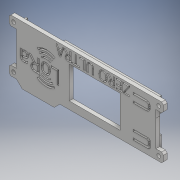
# Autodesk Inventor part: ttgo_lora_oled_case_lid
Saved by Autodesk Inventor 2017 (Build 210142000, 142)
## iProperties
Created: 2021-11-16
Part Number: ttgo_lora_oled_case_lid
Material: Generic
Document SubType Name: Modeling
Designer: simulator
Density: 1 g/cm^3
Appearance: Default
Author: simulator
Autodesk Inventor part; units mm, degrees
ref_plane "YZ Plane" through (0, 0, 0) normal (1, 0, 0) x (0, 1, 0)
ref_plane "XZ Plane" through (0, 0, 0) normal (0, 1, 0) x (-1, 0, 0)
ref_plane "XY Plane" through (0, 0, 0) normal (0, 0, 1) x (1, 0, 0)
sketch "Sketch1" plane through (0, 0, 0) normal (0, 1, 0) x (-1, 0, 0)
  circle A0 centre (-53.5, -14.5) radius 1
  circle A1 centre (23.5, -14.5) radius 1
  circle A2 centre (23.5, 8.5) radius 1
  circle A3 centre (-53.5, 8.5) radius 1
  line L0 (-51, -16) -> (-51, -8)
  line L1 (-51, -8) -> (-52, -8)
  line L2 (-52, -8) -> (-52, -12)
  line L3 (-55, -12) -> (-52, -12)
  line L4 (-56, -13) -> (-55, -12)
  line L5 (-56, -16) -> (-56, -13)
  line L6 (-55, -17) -> (-56, -16)
  line L7 (-1, -17) -> (-55, -17)
  line L8 (-1, -17) -> (2, -20)
  line L9 (2, -20) -> (19, -20)
  line L10 (19, -20) -> (22, -17)
  line L11 (22, -17) -> (25, -17)
  line L12 (25, -17) -> (26, -16)
  line L13 (26, -16) -> (26, -13)
  line L14 (26, -13) -> (25, -12)
  line L15 (25, -12) -> (22, -12)
  line L16 (22, -12) -> (22, 6)
  line L17 (25, 6) -> (22, 6)
  line L18 (26, 7) -> (25, 6)
  line L19 (26, 10) -> (26, 7)
  line L20 (25, 11) -> (26, 10)
  line L21 (-55, 11) -> (25, 11)
  line L22 (-55, 11) -> (-56, 10)
  line L23 (-56, 10) -> (-56, 7)
  line L24 (-56, 7) -> (-55, 6)
  line L25 (-55, 6) -> (-52, 6)
  line L26 (-52, 6) -> (-52, 2)
  line L27 (-52, 2) -> (-51, 2)
  line L28 (-51, 2) -> (-51, 10)
  line L29 (-51, 10) -> (0, 10)
  line L30 (0, 10) -> (0, 2)
  line L31 (0, 2) -> (2.5, 2)
  line L32 (2.5, 2) -> (2.5, 10)
  line L33 (2.5, 10) -> (21, 10)
  line L34 (21, 10) -> (21, -16)
  line L35 (21, -16) -> (2.5, -16)
  line L36 (2.5, -16) -> (2.5, -8)
  line L37 (2.5, -8) -> (0, -8)
  line L38 (0, -8) -> (0, -16)
  line L39 (0, -16) -> (-51, -16)
  point P0 (0, 0)
  point P1 (0, 0)
  constraints: 80 end point, 4 centre point
sketch "Sketch2" plane through (0, 0, 0) normal (0, 1, 0) x (-1, 0, 0)
  line L0 (-33, 2) -> (-33, -13)
  line L1 (-33, -13) -> (-8, -13)
  line L2 (-40, -14) -> (-49, -14)
  line L3 (-49, -9) -> (-40, -9)
  line L4 (-49, -14) -> (-49, -9)
  line L5 (19, -20) -> (2, -20)
  line L6 (-8, -13) -> (-8, 2)
  line L7 (22, -12) -> (22, 6) projected
  line L8 (22, -17) -> (25, -17) projected
  line L9 (25, -17) -> (26, -16) projected
  line L10 (26, -16) -> (26, -13) projected
  line L11 (25, -12) -> (22, -12) projected
  line L12 (-55, -12) -> (-52, -12)
  circle A0 centre (-53.5, -14.5) radius 1
  line L13 (-52, 2) -> (-52, -12)
  line L14 (-52, 6) -> (-52, 2)
  line L15 (-55, 6) -> (-52, 6)
  circle A1 centre (-53.5, 8.5) radius 1
  line L16 (-1, -17) -> (-55, -17)
  line L17 (-55, 11) -> (25, 11)
  circle A2 centre (23.5, 8.5) radius 1
  circle A3 centre (23.5, -14.5) radius 1
  line L18 (-55, -17) -> (-56, -16)
  line L19 (-56, -16) -> (-56, -13)
  line L20 (-56, -13) -> (-55, -12)
  line L21 (-1, -17) -> (2, -20)
  line L22 (2, -20) -> (19, -20)
  line L23 (22, -12) -> (22, 6)
  line L24 (25, 11) -> (26, 10)
  line L25 (26, 10) -> (26, 7)
  line L26 (25, 6) -> (22, 6)
  line L27 (26, 7) -> (25, 6)
  line L28 (19, -20) -> (22, -17)
  line L29 (25, -12) -> (22, -12)
  line L30 (26, -13) -> (25, -12)
  line L31 (22, -17) -> (25, -17)
  line L32 (26, -16) -> (26, -13)
  line L33 (25, -17) -> (26, -16)
  line L34 (-55, 11) -> (-56, 10)
  line L35 (-56, 7) -> (-55, 6)
  line L36 (-56, 10) -> (-56, 7)
  line L37 (-8, 2) -> (-33, 2)
  arc A4 (-52, 1) -> (-52, 2) centre (-420844.4746, 2.0039) ccw
  line L38 (-40, -8) -> (-40, -15)
  line L39 (-38, -13) -> (-48, -13)
  line L40 (-48, -13) -> (-48, -10)
  line L41 (-48, -10) -> (-38, -10)
  line L42 (-38, -10) -> (-38, -13)
  line L43 (22, -3) -> (-52, -3)
  line L44 (-40, -14) -> (-49, -14)
  line L45 (-49, -14) -> (-49, -13)
  line L46 (-49, -13) -> (-40, -13)
  line L47 (-40, -13) -> (-40, -14)
  line L48 (-49, -9) -> (-48, -9)
  line L49 (-48, -9) -> (-48, -14)
  line L50 (-48, -14) -> (-49, -14)
  line L51 (-49, -14) -> (-49, -9)
  line L52 (-49, -9) -> (-40, -9)
  line L53 (-40, -9) -> (-40, -10)
  line L54 (-40, -10) -> (-49, -10)
  line L55 (-49, -10) -> (-49, -9)
  line L56 (-40, -9) -> (-39, -9)
  line L57 (-39, -9) -> (-39, -10)
  line L58 (-39, -10) -> (-40, -10)
  line L59 (-40, -10) -> (-40, -9)
  line L60 (-40, -14) -> (-39, -14)
  line L61 (-39, -14) -> (-39, -13)
  line L62 (-39, -13) -> (-40, -13)
  line L63 (-40, -13) -> (-40, -14)
  line L64 (-49, 3) -> (-40, 3)
  line L65 (-49, 8) -> (-49, 3)
  line L66 (-40, 8) -> (-49, 8)
  line L67 (-40, 2) -> (-40, 9)
  line L68 (-38, 7) -> (-48, 7)
  line L69 (-48, 7) -> (-48, 4)
  line L70 (-48, 4) -> (-38, 4)
  line L71 (-38, 4) -> (-38, 7)
  line L72 (-40, 8) -> (-49, 8)
  line L73 (-49, 8) -> (-49, 7)
  line L74 (-49, 7) -> (-40, 7)
  line L75 (-40, 7) -> (-40, 8)
  line L76 (-49, 3) -> (-48, 3)
  line L77 (-48, 3) -> (-48, 8)
  line L78 (-48, 8) -> (-49, 8)
  line L79 (-49, 8) -> (-49, 3)
  line L80 (-49, 3) -> (-40, 3)
  line L81 (-40, 3) -> (-40, 4)
  line L82 (-40, 4) -> (-49, 4)
  line L83 (-49, 4) -> (-49, 3)
  line L84 (-40, 3) -> (-39, 3)
  line L85 (-39, 3) -> (-39, 4)
  line L86 (-39, 4) -> (-40, 4)
  line L87 (-40, 4) -> (-40, 3)
  line L88 (-40, 8) -> (-39, 8)
  line L89 (-39, 8) -> (-39, 7)
  line L90 (-39, 7) -> (-40, 7)
  line L91 (-40, 7) -> (-40, 8)
  point P0 (-56, 8.5)
  point P1 (-56, -14.5)
  point P2 (-48, -11.5)
  point P3 (-48, -11.5)
  point P4 (-48, 5.5)
  point P5 (-48, 5.5)
  dimension "d1" = 5
  dimension "d2" = 10
  dimension "d3" = 3
  dimension "d4" = 1
  constraints: 174 end point, 27 symmetric about line, 17 point on line, 12 parallel, 11 horizontal, 7 perpendicular, 5 centre point, 3 midpoint, 3 vertical, 2 point on circle, 1 tangent, 7 other
  measures "d1" distance of L4.start L3.start
  measures "d2" distance of L40.end L41.end
  measures "d3" distance of L39.end L40.end
  measures "d4" distance from line of point (-48, -11.5) L4
extrude "Extrusion1" add sketch "Sketch2" along normal blind 2 contours L0 L43 L13 L14 L15 L35 L36 L34 L17 L24 L25 L27 L26 L7 L6 L37 | L0 L1 L6 L43 L7 L11 L30 L10 L9 L8 L28 L5 L21 L16 L18 L19 L20 L12 L13 | L38 L39 L61 L60 | L39 L40 L41 L38 | L38 L41 L42 L39 | L38 L56 L57 L41 | L67 L70 L85 L84 | L69 L68 L67 L70 | L67 L68 L71 L70 | L67 L88 L89 L68
sketch "Sketch3" plane through (0, 2, 0) normal (0, 1, 0) x (1, 0, 0)
  circle A0 centre (53.5, 14.5) radius 1
  circle A1 centre (-23.5, 14.5) radius 1
  circle A2 centre (-23.5, -8.5) radius 1
  circle A3 centre (53.5, -8.5) radius 1
  line L0 (51, 16) -> (51, 8)
  line L1 (51, 8) -> (52, 8)
  line L2 (52, 8) -> (52, 12)
  line L3 (55, 12) -> (52, 12)
  line L4 (56, 13) -> (55, 12)
  line L5 (56, 16) -> (56, 13)
  line L6 (55, 17) -> (56, 16)
  line L7 (1, 17) -> (55, 17)
  line L8 (1, 17) -> (-2, 20)
  line L9 (-2, 20) -> (-19, 20)
  line L10 (-19, 20) -> (-22, 17)
  line L11 (-22, 17) -> (-25, 17)
  line L12 (-25, 17) -> (-26, 16)
  line L13 (-26, 16) -> (-26, 13)
  line L14 (-26, 13) -> (-25, 12)
  line L15 (-25, 12) -> (-22, 12)
  line L16 (-22, 12) -> (-22, -6)
  line L17 (-25, -6) -> (-22, -6)
  line L18 (-26, -7) -> (-25, -6)
  line L19 (-26, -10) -> (-26, -7)
  line L20 (-25, -11) -> (-26, -10)
  line L21 (55, -11) -> (-25, -11)
  line L22 (55, -11) -> (56, -10)
  line L23 (56, -10) -> (56, -7)
  line L24 (56, -7) -> (55, -6)
  line L25 (55, -6) -> (52, -6)
  line L26 (52, -6) -> (52, -2)
  line L27 (52, -2) -> (51, -2)
  line L28 (51, -2) -> (51, -10)
  line L29 (51, -10) -> (0, -10)
  line L30 (0, -10) -> (0, -2)
  line L31 (0, -2) -> (-2.5, -2)
  line L32 (-2.5, -2) -> (-2.5, -10)
  line L33 (-2.5, -10) -> (-21, -10)
  line L34 (-21, -10) -> (-21, 16)
  line L35 (-21, 16) -> (-2.5, 16)
  line L36 (-2.5, 16) -> (-2.5, 8)
  line L37 (-2.5, 8) -> (0, 8)
  line L38 (0, 8) -> (0, 16)
  line L39 (0, 16) -> (51, 16)
  circle A4 centre (-23.5, 14.5) radius 1 projected
  line L40 (0, 16) -> (51, 16)
  line L41 (51, 16) -> (51, 15)
  line L42 (51, 15) -> (0, 15)
  line L43 (0, 15) -> (0, 16)
  line L44 (0, -10) -> (51, -10)
  line L45 (51, -10) -> (51, -9)
  line L46 (51, -9) -> (0, -9)
  line L47 (0, -9) -> (0, -10)
  line L48 (-21, 16) -> (-20, 16)
  line L49 (-20, 16) -> (-20, -10)
  line L50 (-20, -10) -> (-21, -10)
  line L51 (-21, -10) -> (-21, 16)
  line L52 (51, -2) -> (50, -2)
  line L53 (50, -2) -> (50, -10)
  line L54 (50, -10) -> (51, -10)
  line L55 (51, -10) -> (51, -2)
  line L56 (51, 8) -> (50, 8)
  line L57 (50, 8) -> (50, 16)
  line L58 (50, 16) -> (51, 16)
  line L59 (51, 16) -> (51, 8)
  point P0 (0, 0)
  point P1 (0, 0)
  dimension "d8" = 1
  dimension "d9" = 1
  dimension "d10" = 1
  dimension "d11" = 1
  constraints: 120 end point, 10 parallel, 6 point on line, 5 horizontal, 5 perpendicular, 4 centre point
  measures "d8" distance of L40.end L41.end
  measures "d9" distance of L45.end L44.end
  measures "d10" distance of L49.end L50.end
  measures "d11" distance of L54.end L53.end
extrude "Extrusion2" add sketch "Sketch3" along normal blind 2 contours L0 L42 L57 L39 | L0 L56 L57 L42 | L57 L42 L38 L39 | L49 L33 L34 L35 | L46 L53 L29 L30 | L53 L52 L28 L46 | L46 L28 L29 L53
chamfer "Chamfer1" distance 1 angle 45 3 edges at (-20, 2, -3) (25, 2, -15) (25, 2, 9)
fillet "Fillet1" radius 1 3 edges at (48, 1, -13) (48, 1, 4) (48, 1, 7)
fillet "Fillet2" radius 1 3 edges at (49, 1, -14) (49, 1, -9) (48, 1, -10)
sketch "Sketch4" plane through (0, 0, 0) normal (0, -1, 0) x (1, 0, 0)
  line L0 (48, -14) -> (40, -14) projected
  line L1 (40, -13) -> (40, -14) projected
  line L2 (47, -13) -> (40, -13) projected
  arc A0 (47, -13) -> (48, -12) centre (47, -12) ccw projected
  line L3 (48, -12) -> (48, -11) projected
  line L4 (47, -10) -> (40, -10) projected
  line L5 (40, -10) -> (40, -9) projected
  line L6 (40, -9) -> (48, -9) projected
  arc A1 (48, 6) -> (47, 7) centre (47, 6) ccw projected
  line L7 (47, 7) -> (40, 7) projected
  line L8 (40, 7) -> (40, 8) projected
  line L9 (40, 8) -> (49, 8) projected
  line L10 (49, 8) -> (49, 3) projected
  line L11 (49, 3) -> (40, 3) projected
  line L12 (40, 3) -> (40, 4) projected
  line L13 (40, 4) -> (47, 4) projected
  arc A2 (47, 4) -> (48, 5) centre (47, 5) ccw projected
  line L14 (48, 5) -> (48, 6) projected
  line L15 (-22, -17) -> (-19, -20) projected
  line L16 (-19, -20) -> (-2, -20) projected
  line L17 (-2, -20) -> (1, -17) projected
  line L18 (1, -17) -> (55, -17) projected
  line L19 (55, -17) -> (56, -16) projected
  line L20 (56, -16) -> (56, -13) projected
  line L21 (56, -13) -> (55, -12) projected
  line L22 (55, -12) -> (52, -12) projected
  line L23 (52, -12) -> (52, 2) projected
  line L24 (52, 2) -> (52, 6) projected
  line L25 (52, 6) -> (55, 6) projected
  line L26 (55, 6) -> (56, 7) projected
  line L27 (56, 7) -> (56, 10) projected
  line L28 (56, 10) -> (55, 11) projected
  line L29 (55, 11) -> (-25, 11) projected
  line L30 (-25, 11) -> (-26, 10) projected
  line L31 (-26, 10) -> (-26, 7) projected
  line L32 (-26, 7) -> (-25, 6) projected
  line L33 (-25, 6) -> (-22, 6) projected
  line L34 (-22, 6) -> (-22, -12) projected
  line L35 (-22, -12) -> (-25, -12) projected
  line L36 (-25, -12) -> (-26, -13) projected
  line L37 (-26, -13) -> (-26, -16) projected
  line L38 (-26, -16) -> (-25, -17) projected
  line L39 (-25, -17) -> (-22, -17) projected
  circle A3 centre (53.5, -14.5) radius 1 projected
  circle A4 centre (53.5, 8.5) radius 1 projected
  circle A5 centre (-23.5, 8.5) radius 1 projected
  circle A6 centre (-23.5, -14.5) radius 1 projected
  line L40 (33, 2) -> (33, -13) projected
  line L41 (33, -13) -> (8, -13) projected
  line L42 (8, -13) -> (8, 2) projected
  line L43 (8, 2) -> (33, 2) projected
  line L44 (33, 2) -> (8, 2)
  line L45 (8, 2) -> (8, 4)
  line L46 (8, 4) -> (33, 4)
  line L47 (33, 4) -> (33, 2)
  line L48 (8, -13) -> (6, -13)
  line L49 (6, -13) -> (6, 4)
  line L50 (6, 4) -> (8, 4)
  line L51 (8, 4) -> (8, -13)
  arc A7 (48, -11) -> (47, -10) centre (47, -11) ccw projected
  arc A8 (49, -10) -> (48, -9) centre (48, -10) ccw projected
  line L52 (49, -10) -> (49, -13) projected
  arc A9 (48, -14) -> (49, -13) centre (48, -13) ccw projected
  point P0 (0, 0)
  dimension "d19" = 2
  dimension "d20" = 2
  constraints: 16 end point, 4 parallel, 2 horizontal, 2 perpendicular, 1 point on line
  measures "d19" distance of L44.end L45.end
  measures "d20" distance of L49.end L50.end
extrude "Extrusion3" cut sketch "Sketch4" against normal blind 10 contours L43 L45 L46 L47 | L42 L48 L49 L50 L45
fillet "Fillet3" radius 2 2 edges at (49, 1, 8) (49, 1, 3)
sketch "Sketch5" plane through (0, 0, 0) normal (0, -1, 0) x (1, 0, 0)
  line L0 (1.2295, -8.816) -> (-31.2797, -8.816) construction
  line L1 (-31.2797, -8.816) -> (-31.2797, 0.8087) construction
  line L2 (-31.2797, 0.8087) -> (1.2295, 0.8087) construction
  line L3 (1.2295, 0.8087) -> (1.2295, -8.816) construction
  line L4 (-3.9903, -0.4302) -> (-3.6005, 0.1309)
  line L5 (-3.0082, 0.9561) -> (-2.5783, 1.563)
  line L6 (-2.0871, 2.2564) -> (-1.495, 3.0924)
  arc A0 (-3.9903, -0.4302) -> (-8.565, -0.5063) centre (-6.2185, -4.0213) ccw
  arc A1 (-8.6056, -7.5089) -> (-4.0659, -7.6583) centre (-6.2185, -4.0213) ccw
  arc A2 (-3.6005, 0.1309) -> (-8.9501, 0.0571) centre (-6.2185, -4.0213) ccw
  arc A3 (-8.9329, -7.9708) -> (-3.7378, -8.1216) centre (-6.2185, -4.0213) ccw
  line L7 (-8.565, -0.5063) -> (-8.9501, 0.0571)
  arc A4 (-3.0082, 0.9561) -> (-9.5252, 0.8926) centre (-6.2185, -4.0213) ccw
  arc A5 (-9.5865, -8.8935) -> (-3.0831, -9.0463) centre (-6.2185, -4.0213) ccw
  arc A6 (-2.5783, 1.563) -> (-9.9458, 1.5053) centre (-6.2185, -4.0213) ccw
  arc A7 (-10.016, -9.4999) -> (-2.6531, -9.6537) centre (-6.2185, -4.0213) ccw
  arc A8 (-2.0871, 2.2564) -> (-10.4264, 2.2054) centre (-6.2185, -4.0213) ccw
  arc A9 (-1.495, 3.0924) -> (-11.0059, 3.0495) centre (-6.2185, -4.0213) ccw
  line L8 (-9.5252, 0.8926) -> (-9.9458, 1.5053)
  line L9 (-10.4264, 2.2054) -> (-11.0059, 3.0495)
  line L10 (-4.0659, -7.6583) -> (-3.7378, -8.1216)
  line L11 (-2.6531, -9.6537) -> (-3.0831, -9.0463)
  line L12 (-2.1618, -10.3476) -> (-1.5696, -11.184)
  arc A10 (-11.9743, 0.8087) -> (-12.0038, -8.816) centre (-6.2185, -4.0213) ccw
  line L13 (-10.5069, -10.1929) -> (-11.0988, -11.0284)
  arc A11 (-13.2592, 0.8087) -> (-13.2833, -8.816) centre (-6.2185, -4.0213) ccw
  line L14 (-8.6056, -7.5089) -> (-8.9329, -7.9708)
  line L15 (-9.5865, -8.8935) -> (-10.016, -9.4999)
  arc A12 (-10.5069, -10.1929) -> (-2.1618, -10.3476) centre (-6.2185, -4.0213) ccw
  arc A13 (-0.4333, -8.816) -> (-0.4627, 0.8087) centre (-6.2185, -4.0213) ccw
  arc A14 (-11.0988, -11.0284) -> (-1.5696, -11.184) centre (-6.2185, -4.0213) ccw
  arc A15 (0.8463, -8.816) -> (0.8222, 0.8087) centre (-6.2185, -4.0213) ccw
  line L16 (38.3682, 4.8239) -> (-10.0254, 4.8239) construction
  line L17 (-10.0254, 4.8239) -> (-10.0254, 15.0346) construction
  line L18 (-10.0254, 15.0346) -> (38.3682, 15.0346) construction
  line L19 (38.3682, 15.0346) -> (38.3682, 4.8239) construction
  line L20 (34.6729, 9.9292) -> (38.1656, 9.9292)
  line L21 (38.1656, 9.9292) -> (38.1656, 9.3093)
  line L22 (38.1656, 9.3093) -> (35.4914, 5.5208)
  line L23 (35.4914, 5.5208) -> (38.0441, 5.5208)
  line L24 (38.0441, 5.5208) -> (38.0441, 4.9292)
  line L25 (38.0441, 4.9292) -> (34.7418, 4.9292)
  line L26 (34.7418, 4.9292) -> (34.7418, 5.5289)
  line L27 (34.7418, 5.5289) -> (37.4444, 9.3377)
  line L28 (37.4444, 9.3377) -> (34.6729, 9.3377)
  line L29 (34.6729, 9.3377) -> (34.6729, 9.9292)
  line L30 (34.0165, 9.9292) -> (34.0165, 4.9292)
  line L31 (34.0165, 4.9292) -> (30.8885, 4.9292)
  line L32 (30.8885, 4.9292) -> (30.8885, 5.5208)
  line L33 (30.8885, 5.5208) -> (33.352, 5.5208)
  line L34 (33.352, 5.5208) -> (33.352, 6.8903)
  line L35 (33.352, 6.8903) -> (31.0546, 6.8903)
  line L36 (31.0546, 6.8903) -> (31.0546, 7.4819)
  line L37 (31.0546, 7.4819) -> (33.352, 7.4819)
  line L38 (33.352, 7.4819) -> (33.352, 9.3377)
  line L39 (33.352, 9.3377) -> (30.8885, 9.3377)
  line L40 (30.8885, 9.3377) -> (30.8885, 9.9292)
  line L41 (30.8885, 9.9292) -> (34.0165, 9.9292)
  line L42 (26.2896, 9.9292) -> (27.1527, 9.9292)
  line L43 (27.1527, 9.9292) -> (28.7329, 7.9398)
  line L44 (28.7329, 7.9398) -> (29.4946, 7.9398)
  line L45 (29.4946, 7.9398) -> (29.4946, 9.9292)
  line L46 (29.4946, 9.9292) -> (30.1591, 9.9292)
  line L47 (30.1591, 9.9292) -> (30.1591, 4.9292)
  line L48 (30.1591, 4.9292) -> (28.8707, 4.9292)
  spline S0 degree 2 poles (28.8707, 4.9292) (28.4412, 4.9292) (27.8617, 5.0224) (27.5984, 5.1926) knots 0 0 0 1 2 2 2
  spline S1 degree 2 poles (27.5984, 5.1926) (27.335, 5.3628) (27.0311, 5.8936) (27.0311, 6.2866) knots 0 0 0 1 2 2 2
  spline S2 degree 2 poles (27.0311, 6.2866) (27.0311, 6.8336) (27.5903, 7.5751) (28.0684, 7.7534) knots 0 0 0 1 2 2 2
  line L49 (28.0684, 7.7534) -> (26.2896, 9.9292)
  spline S3 degree 2 poles (27.724, 6.3393) (27.724, 6.1205) (27.8779, 5.7842) (28.04, 5.6748) knots 0 0 0 1 2 2 2
  spline S4 degree 2 poles (28.04, 5.6748) (28.1818, 5.5816) (28.5587, 5.5046) (28.8342, 5.5046) knots 0 0 0 1 2 2 2
  line L50 (28.8342, 5.5046) -> (29.4946, 5.5046)
  line L51 (29.4946, 5.5046) -> (29.4946, 7.3847)
  line L52 (29.4946, 7.3847) -> (28.9112, 7.3847)
  spline S5 degree 2 poles (28.9112, 7.3847) (28.6235, 7.3847) (28.1656, 7.2834) (28.0076, 7.1254) knots 0 0 0 1 2 2 2
  spline S6 degree 2 poles (28.0076, 7.1254) (27.8617, 6.9876) (27.724, 6.5986) (27.724, 6.3393) knots 0 0 0 1 2 2 2
  spline S7 degree 2 poles (22.3553, 5.5006) (22.0716, 5.8328) (21.7556, 6.8053) (21.7556, 7.4292) knots 0 0 0 1 2 2 2
  spline S8 degree 2 poles (21.7556, 7.4292) (21.7556, 8.037) (22.0635, 9.0216) (22.3553, 9.3539) knots 0 0 0 1 2 2 2
  spline S9 degree 2 poles (22.3553, 9.3539) (22.6632, 9.7023) (23.4776, 10.0346) (23.9679, 10.0346) knots 0 0 0 1 2 2 2
  spline S10 degree 2 poles (23.9679, 10.0346) (24.4744, 10.0346) (25.2848, 9.6902) (25.5805, 9.3539) knots 0 0 0 1 2 2 2
  spline S11 degree 2 poles (25.5805, 9.3539) (25.8682, 9.0216) (26.1762, 8.0451) (26.1762, 7.4292) knots 0 0 0 1 2 2 2
  spline S12 degree 2 poles (26.1762, 7.4292) (26.1762, 6.8012) (25.8642, 5.845) (25.5765, 5.5006) knots 0 0 0 1 2 2 2
  spline S13 degree 2 poles (25.5765, 5.5006) (25.2848, 5.1683) (24.4703, 4.8239) (23.9679, 4.8239) knots 0 0 0 1 2 2 2
  spline S14 degree 2 poles (23.9679, 4.8239) (23.4574, 4.8239) (22.6389, 5.1805) (22.3553, 5.5006) knots 0 0 0 1 2 2 2
  spline S15 degree 2 poles (22.4485, 7.4292) (22.4485, 6.9349) (22.6632, 6.1691) (22.8577, 5.9179) knots 0 0 0 1 2 2 2
  spline S16 degree 2 poles (22.8577, 5.9179) (23.0562, 5.6586) (23.6154, 5.3993) (23.9638, 5.3993) knots 0 0 0 1 2 2 2
  spline S17 degree 2 poles (23.9638, 5.3993) (24.3245, 5.3993) (24.8674, 5.6505) (25.0741, 5.9179) knots 0 0 0 1 2 2 2
  spline S18 degree 2 poles (25.0741, 5.9179) (25.2726, 6.1732) (25.4833, 6.943) (25.4833, 7.4292) knots 0 0 0 1 2 2 2
  spline S19 degree 2 poles (25.4833, 7.4292) (25.4833, 8.4139) (24.6567, 9.4592) (23.9638, 9.4592) knots 0 0 0 1 2 2 2
  spline S20 degree 2 poles (23.9638, 9.4592) (23.271, 9.4592) (22.4485, 8.4139) (22.4485, 7.4292) knots 0 0 0 1 2 2 2
  spline S21 degree 2 poles (17.1324, 10.0346) (17.5741, 10.0346) (18.2305, 9.8036) (18.4614, 9.5727) knots 0 0 0 1 2 2 2
  spline S22 degree 2 poles (18.4614, 9.5727) (18.7248, 9.3134) (18.9395, 8.584) (18.9395, 8.0492) knots 0 0 0 1 2 2 2
  line L53 (18.9395, 8.0492) -> (18.9395, 4.9292)
  line L54 (18.9395, 4.9292) -> (18.275, 4.9292)
  line L55 (18.275, 4.9292) -> (18.275, 8.0492)
  spline S23 degree 2 poles (18.275, 8.0492) (18.275, 8.3976) (18.1859, 8.8677) (18.0603, 9.0581) knots 0 0 0 1 2 2 2
  spline S24 degree 2 poles (18.0603, 9.0581) (17.9266, 9.2607) (17.4647, 9.4673) (17.1324, 9.4673) knots 0 0 0 1 2 2 2
  spline S25 degree 2 poles (17.1324, 9.4673) (16.8204, 9.4673) (16.3342, 9.2607) (16.2005, 9.0581) knots 0 0 0 1 2 2 2
  spline S26 degree 2 poles (16.2005, 9.0581) (16.0749, 8.8677) (15.9857, 8.4017) (15.9857, 8.0654) knots 0 0 0 1 2 2 2
  line L56 (15.9857, 8.0654) -> (15.9857, 4.9292)
  line L57 (15.9857, 4.9292) -> (15.3212, 4.9292)
  line L58 (15.3212, 4.9292) -> (15.3212, 8.0492)
  spline S27 degree 2 poles (15.3212, 8.0492) (15.3212, 8.5719) (15.5319, 9.3174) (15.7993, 9.5727) knots 0 0 0 1 2 2 2
  spline S28 degree 2 poles (15.7993, 9.5727) (16.0384, 9.8077) (16.6705, 10.0346) (17.1324, 10.0346) knots 0 0 0 1 2 2 2
  line L59 (11.472, 9.9292) -> (14.369, 9.9292)
  line L60 (14.369, 9.9292) -> (14.369, 4.9292)
  line L61 (14.369, 4.9292) -> (13.7045, 4.9292)
  line L62 (13.7045, 4.9292) -> (13.7045, 9.3377)
  line L63 (13.7045, 9.3377) -> (11.472, 9.3377)
  line L64 (11.472, 9.3377) -> (11.472, 9.9292)
  line L65 (9.7823, 9.9292) -> (9.7823, 5.5208)
  line L66 (9.7823, 5.5208) -> (11.4598, 5.5208)
  line L67 (11.4598, 5.5208) -> (11.4598, 4.9292)
  line L68 (11.4598, 4.9292) -> (7.4403, 4.9292)
  line L69 (7.4403, 4.9292) -> (7.4403, 5.5208)
  line L70 (7.4403, 5.5208) -> (9.1178, 5.5208)
  line L71 (9.1178, 5.5208) -> (9.1178, 9.9292)
  line L72 (9.1178, 9.9292) -> (9.7823, 9.9292)
  line L73 (3.0643, 9.9292) -> (3.9274, 9.9292)
  line L74 (3.9274, 9.9292) -> (5.5076, 7.9398)
  line L75 (5.5076, 7.9398) -> (6.2694, 7.9398)
  line L76 (6.2694, 7.9398) -> (6.2694, 9.9292)
  line L77 (6.2694, 9.9292) -> (6.9339, 9.9292)
  line L78 (6.9339, 9.9292) -> (6.9339, 4.9292)
  line L79 (6.9339, 4.9292) -> (5.6454, 4.9292)
  spline S29 degree 2 poles (5.6454, 4.9292) (5.2159, 4.9292) (4.6365, 5.0224) (4.3731, 5.1926) knots 0 0 0 1 2 2 2
  spline S30 degree 2 poles (4.3731, 5.1926) (4.1097, 5.3628) (3.8058, 5.8936) (3.8058, 6.2866) knots 0 0 0 1 2 2 2
  spline S31 degree 2 poles (3.8058, 6.2866) (3.8058, 6.8336) (4.365, 7.5751) (4.8431, 7.7534) knots 0 0 0 1 2 2 2
  line L80 (4.8431, 7.7534) -> (3.0643, 9.9292)
  spline S32 degree 2 poles (4.4987, 6.3393) (4.4987, 6.1205) (4.6527, 5.7842) (4.8147, 5.6748) knots 0 0 0 1 2 2 2
  spline S33 degree 2 poles (4.8147, 5.6748) (4.9566, 5.5816) (5.3334, 5.5046) (5.6089, 5.5046) knots 0 0 0 1 2 2 2
  line L81 (5.6089, 5.5046) -> (6.2694, 5.5046)
  line L82 (6.2694, 5.5046) -> (6.2694, 7.3847)
  line L83 (6.2694, 7.3847) -> (5.6859, 7.3847)
  spline S34 degree 2 poles (5.6859, 7.3847) (5.3982, 7.3847) (4.9403, 7.2834) (4.7823, 7.1254) knots 0 0 0 1 2 2 2
  spline S35 degree 2 poles (4.7823, 7.1254) (4.6365, 6.9876) (4.4987, 6.5986) (4.4987, 6.3393) knots 0 0 0 1 2 2 2
  line L84 (3.2062, 9.9292) -> (1.5206, 4.9292)
  line L85 (1.5206, 4.9292) -> (0.7021, 4.9292)
  line L86 (0.7021, 4.9292) -> (-0.9835, 9.9292)
  line L87 (-0.9835, 9.9292) -> (-0.2825, 9.9292)
  line L88 (-0.2825, 9.9292) -> (0.1713, 8.5314)
  line L89 (0.1713, 8.5314) -> (2.0797, 8.5314)
  line L90 (2.0797, 8.5314) -> (2.5335, 9.9292)
  line L91 (2.5335, 9.9292) -> (3.2062, 9.9292)
  line L92 (0.3536, 7.9641) -> (1.1275, 5.61)
  line L93 (1.1275, 5.61) -> (1.8974, 7.9641)
  line L94 (1.8974, 7.9641) -> (0.3536, 7.9641)
  line L95 (-3.7002, -1.574) -> (0.4959, -1.574)
  line L96 (0.4959, -1.574) -> (0.4959, -8.816)
  line L97 (0.4959, -8.816) -> (-0.4665, -8.816)
  line L98 (-0.4665, -8.816) -> (-0.4665, -2.4309)
  line L99 (-0.4665, -2.4309) -> (-3.7002, -2.4309)
  line L100 (-3.7002, -2.4309) -> (-3.7002, -1.574)
  spline S36 degree 2 poles (-8.8529, -4.2912) (-8.8529, -2.918) (-7.5325, -1.4214) (-6.4291, -1.4214) knots 0 0 0 1 2 2 2
  spline S37 degree 2 poles (-6.4291, -1.4214) (-5.2965, -1.4214) (-3.9995, -2.9649) (-3.9995, -4.2912) knots 0 0 0 1 2 2 2
  spline S38 degree 2 poles (-3.9995, -4.2912) (-3.9995, -5.6528) (-5.3376, -7.161) (-6.4291, -7.161) knots 0 0 0 1 2 2 2
  spline S39 degree 2 poles (-6.4291, -7.161) (-7.5325, -7.161) (-8.8529, -5.6587) (-8.8529, -4.2912) knots 0 0 0 1 2 2 2
  spline S40 degree 2 poles (-7.9081, -4.2912) (-7.9081, -5.3476) (-7.1393, -6.3746) (-6.4291, -6.3746) knots 0 0 0 1 2 2 2
  spline S41 degree 2 poles (-6.4291, -6.3746) (-5.719, -6.3746) (-4.9444, -5.3476) (-4.9444, -4.2912) knots 0 0 0 1 2 2 2
  spline S42 degree 2 poles (-4.9444, -4.2912) (-4.9444, -3.2642) (-5.719, -2.2078) (-6.4291, -2.2078) knots 0 0 0 1 2 2 2
  spline S43 degree 2 poles (-6.4291, -2.2078) (-7.1334, -2.2078) (-7.9081, -3.2466) (-7.9081, -4.2912) knots 0 0 0 1 2 2 2
  line L101 (-15.467, -1.574) -> (-14.2169, -1.574)
  line L102 (-14.2169, -1.574) -> (-11.9281, -4.4556)
  line L103 (-11.9281, -4.4556) -> (-10.8248, -4.4556)
  line L104 (-10.8248, -4.4556) -> (-10.8248, -1.574)
  line L105 (-10.8248, -1.574) -> (-9.8623, -1.574)
  line L106 (-9.8623, -1.574) -> (-9.8623, -8.816)
  line L107 (-9.8623, -8.816) -> (-11.7286, -8.816)
  spline S44 degree 2 poles (-11.7286, -8.816) (-12.3507, -8.816) (-13.1899, -8.681) (-13.5714, -8.4346) knots 0 0 0 1 2 2 2
  spline S45 degree 2 poles (-13.5714, -8.4346) (-13.9528, -8.1881) (-14.393, -7.4193) (-14.393, -6.85) knots 0 0 0 1 2 2 2
  spline S46 degree 2 poles (-14.393, -6.85) (-14.393, -6.0577) (-13.5831, -4.9838) (-12.8906, -4.7255) knots 0 0 0 1 2 2 2
  line L108 (-12.8906, -4.7255) -> (-15.467, -1.574)
  spline S47 degree 2 poles (-13.3894, -6.7737) (-13.3894, -7.0906) (-13.1664, -7.5777) (-12.9317, -7.7362) knots 0 0 0 1 2 2 2
  spline S48 degree 2 poles (-12.9317, -7.7362) (-12.7263, -7.8712) (-12.1805, -7.9827) (-11.7814, -7.9827) knots 0 0 0 1 2 2 2
  line L109 (-11.7814, -7.9827) -> (-10.8248, -7.9827)
  line L110 (-10.8248, -7.9827) -> (-10.8248, -5.2596)
  line L111 (-10.8248, -5.2596) -> (-11.6699, -5.2596)
  spline S49 degree 2 poles (-11.6699, -5.2596) (-12.0866, -5.2596) (-12.7498, -5.4063) (-12.9786, -5.6352) knots 0 0 0 1 2 2 2
  spline S50 degree 2 poles (-12.9786, -5.6352) (-13.1899, -5.8347) (-13.3894, -6.3981) (-13.3894, -6.7737) knots 0 0 0 1 2 2 2
  spline S51 degree 2 poles (-18.9999, -2.1492) (-18.8884, -2.067) (-18.5128, -1.7736) (-18.3368, -1.6855) knots 0 0 0 1 2 2 2
  spline S52 degree 2 poles (-18.3368, -1.6855) (-18.0962, -1.5564) (-17.6443, -1.4214) (-17.2335, -1.4214) knots 0 0 0 1 2 2 2
  spline S53 degree 2 poles (-17.2335, -1.4214) (-16.8989, -1.4214) (-16.2945, -1.6738) (-16.0656, -1.9027) knots 0 0 0 1 2 2 2
  spline S54 degree 2 poles (-16.0656, -1.9027) (-15.8484, -2.1257) (-15.5843, -2.783) (-15.5843, -3.1468) knots 0 0 0 1 2 2 2
  spline S55 degree 2 poles (-15.5843, -3.1468) (-15.5843, -3.7102) (-16.0597, -4.5084) (-16.5762, -4.7373) knots 0 0 0 1 2 2 2
  spline S56 degree 2 poles (-16.5762, -4.7373) (-17.0339, -4.9485) (-18.2781, -5.107) (-18.9999, -5.1481) knots 0 0 0 1 2 2 2
  line L112 (-18.9999, -5.1481) -> (-18.9999, -5.3241)
  spline S57 degree 2 poles (-18.9999, -5.3241) (-18.9999, -5.6411) (-18.8063, -6.0343) (-18.6302, -6.1458) knots 0 0 0 1 2 2 2
  spline S58 degree 2 poles (-18.6302, -6.1458) (-18.4541, -6.2573) (-17.9494, -6.3277) (-17.6795, -6.3277) knots 0 0 0 1 2 2 2
  spline S59 degree 2 poles (-17.6795, -6.3277) (-17.3626, -6.3277) (-16.5057, -6.1399) (-16.0773, -5.958) knots 0 0 0 1 2 2 2
  line L113 (-16.0773, -5.958) -> (-16.0245, -5.958)
  line L114 (-16.0245, -5.958) -> (-16.0245, -6.8911)
  spline S60 degree 2 poles (-16.0245, -6.8911) (-16.2769, -6.9615) (-17.2217, -7.1376) (-17.6853, -7.1376) knots 0 0 0 1 2 2 2
  spline S61 degree 2 poles (-17.6853, -7.1376) (-18.2487, -7.1376) (-19.0175, -6.9615) (-19.3227, -6.7326) knots 0 0 0 1 2 2 2
  spline S62 degree 2 poles (-19.3227, -6.7326) (-19.622, -6.5096) (-19.9155, -5.7995) (-19.9155, -5.2889) knots 0 0 0 1 2 2 2
  line L115 (-19.9155, -5.2889) -> (-19.9155, -1.574)
  line L116 (-19.9155, -1.574) -> (-18.9999, -1.574)
  line L117 (-18.9999, -1.574) -> (-18.9999, -2.1492)
  line L118 (-18.9999, -2.9121) -> (-18.9999, -4.4204)
  spline S63 degree 2 poles (-18.9999, -4.4204) (-18.6713, -4.391) (-17.6795, -4.2912) (-17.3684, -4.1973) knots 0 0 0 1 2 2 2
  spline S64 degree 2 poles (-17.3684, -4.1973) (-17.0046, -4.0858) (-16.5292, -3.6222) (-16.5292, -3.2114) knots 0 0 0 1 2 2 2
  spline S65 degree 2 poles (-16.5292, -3.2114) (-16.5292, -2.7419) (-17.0574, -2.2665) (-17.5621, -2.2665) knots 0 0 0 1 2 2 2
  spline S66 degree 2 poles (-17.5621, -2.2665) (-17.9905, -2.2665) (-18.6948, -2.6363) (-18.9999, -2.9121) knots 0 0 0 1 2 2 2
  point P0 (0, 0)
  constraints: 32 point on circle, 24 end point, 16 centre point, 8 point on line, 5 coincident, 4 other
extrude "Extrusion5" cut sketch "Sketch5" against normal blind 1 contours A0 L7 A2 L4 | A4 L8 A6 L5 | A8 L9 A9 L6 | A1 L10 A3 L14 | A5 L11 A7 L15 | L12 A14 L13 A12 | L102 L103 L104 L105 L106 L107 S44 A10 S48 L109 L110 L111 S49 S50 S46 L108 | A10 L108 A11 L101 L102 | A10 S50 S47 S48 S44 A11 S46 | L108 L101 A11 | A11 S44 S45 S46 | L97 L98 L99 L100 L95 L96 A13 | A13 L96 L97 | L20 L21 L22 L23 L24 L25 L26 L27 L28 L29 | L30 L31 L32 L33 L34 L35 L36 L37 L38 L39 L40 L41 | L42 L43 L44 L45 L46 L47 L48 S0 S1 S2 L49 | S7 S8 S9 S10 S11 S12 S13 S14 | S21 S22 L53 L54 L55 S23 S24 S25 S26 L56 L57 L58 S27 S28 | L59 L60 L61 L62 L63 L64 | L65 L66 L67 L68 L69 L70 L71 L72 | L73 L84 L80 | L80 L84 L85 L86 L87 L88 L89 L90 L91 | L73 L74 L75 L76 L77 L78 L79 S29 S30 S31 L80 L84 | S36 S37 S38 S39 | S51 S52 S53 S54 S55 S56 L112 S57 S58 S59 L113 L114 S60 S61 S62 L115 L116 L117
body "Solid1"
